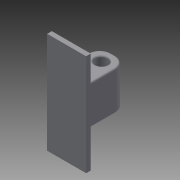
# Autodesk Inventor part: ESP_DISP_LG
Saved by Autodesk Inventor 2015 (Build 190159000, 159)
## iProperties
Created: 2018-04-04
Part Number: ESP_DISP_LG
Material: Типовые
Document SubType Name: Modeling
Designer: JOK
Density: 1 g/cm^3
Appearance: По умолчанию
Author: JOK
Autodesk Inventor part; units mm, degrees
ref_plane "YZ Plane" through (0, 0, 0) normal (1, 0, 0) x (0, 1, 0)
ref_plane "XZ Plane" through (0, 0, 0) normal (0, 1, 0) x (-1, 0, 0)
ref_plane "XY Plane" through (0, 0, 0) normal (0, 0, 1) x (1, 0, 0)
sketch "Эскиз1" plane through (0, 0, 0) normal (0, 1, 0) x (-1, 0, 0)
  line L0 (3.5, 13) -> (-3.5, 13)
  line L1 (-3.5, 13) -> (-3.5, 3)
  line L2 (-3.5, 3) -> (3.5, 3)
  line L3 (3.5, 3) -> (3.5, 13)
  line L4 (3.5, 13) -> (-3.5, 3) construction
  line L5 (-3.5, 13) -> (3.5, 3) construction
  line L6 (5, 21) -> (-5, 21)
  line L7 (-5, 21) -> (-5, -5)
  line L8 (-5, -5) -> (5, -5)
  line L9 (5, -5) -> (5, 21)
  line L10 (5, 21) -> (-5, -5) construction
  line L11 (-5, 21) -> (5, -5) construction
  point P0 (0, 0)
  point P1 (0, 8)
  point P2 (0, 8)
  dimension "d0" = 7
  dimension "d1" = 10
  constraints: 24 end point, 5 midpoint, 4 parallel, 2 horizontal, 2 perpendicular
  measures "d0" distance of L2.end L1.end
  measures "d1" distance of L1.end L0.end
extrude "Выдавливание1" add sketch "Эскиз1" along normal blind 2 contours L3 L2 L1 L0 | L9 L8 L7 L6
sketch "Эскиз2" plane through (0, 2, 0) normal (0, 1, 0) x (1, 0, 0)
  line L0 (-5, -21) -> (5, -21) projected
  line L1 (5, -21) -> (5, 5) projected
  line L2 (5, 5) -> (-5, 5) projected
  line L3 (-5, 5) -> (-5, -21) projected
  point P0 (0, 0)
chamfer "Фаска1" distance 1.4 angle 30 4 edges at (0, 2, 21) (5, 2, 8) (0, 2, -5) (-5, 2, 8) measured on face at (0, 2, -4.5) measured on face at (-4.5, 2, 8) measured on face at (0, 2, 20.5) measured on face at (4.5, 2, 8)
sketch "Эскиз3" plane through (0, 2, 0) normal (0, 1, 0) x (1, 0, 0)
  line L0 (-3.5, -13) -> (3.5, -13)
  line L1 (3.5, -13) -> (3.5, -3)
  line L2 (3.5, -3) -> (-3.5, -3)
  line L3 (-3.5, -3) -> (-3.5, -13)
  line L4 (-3.5, -13) -> (3.5, -3) construction
  line L5 (3.5, -13) -> (-3.5, -3) construction
  point P0 (0, 0)
  point P1 (0, -8)
  dimension "d7" = 7
  constraints: 12 end point, 2 midpoint, 2 parallel, 1 horizontal, 1 perpendicular
  measures "d7" distance of L2.end L1.end
extrude "Выдавливание2" add sketch "Эскиз3" along normal blind 10
fillet "Сопряжение1" radius 3 2 edges at (3.5, 12, 8) (-3.5, 12, 8)
sketch "Эскиз4" plane through (3.5, 2, 3) normal (0, 0, -1) x (-1, 0, 0)
  line L0 (3, 10) -> (4, 10) projected
  line L1 (3.5, 10) -> (3.5, 7)
  circle A0 centre (3.5, 7) radius 1.6
  point P0 (3.5, -2)
  dimension "d11" = 3
  dimension "d12" = 3.2
  constraints: 2 end point, 1 centre point, 1 coincident, 1 midpoint, 1 vertical
  measures "d11" distance of L1.start L1.end
  measures "d12" diameter of A0
extrude "Выдавливание3" cut sketch "Эскиз4" against normal blind 10
fillet "Сопряжение2" radius 0.4 2 edges at (1.6, 9, 3) (1.6, 9, 13)
fillet "Сопряжение3" radius 0.4 10 edges at (3.5, 5.5, 13) (0, 12, 13) (-2.6213, 11.1213, 13) (-3.5, 5.5, 13) (2.6213, 11.1213, 13) (0, 12, 3) (-2.6213, 11.1213, 3) (-3.5, 5.5, 3) (3.5, 5.5, 3) (2.6213, 11.1213, 3)
